Autodesk Fusion 360 part; units mm, degrees
(part 3 of 8)
  spline S62 degree 5 poles (147.1509, -702.208) (147.1492, -702.1152) (147.1456, -701.9297) (147.1398, -701.6516) (147.1309, -701.281) (147.1182, -700.8181) (147.1039, -700.3557) (147.0878, -699.8936) (147.0701, -699.4319) (147.0506, -698.9707) (147.0295, -698.5098) (147.0066, -698.0494) (146.982, -697.5895) (146.9557, -697.13) (146.9276, -696.6709) (146.8978, -696.2123) (146.8662, -695.7542) (146.8328, -695.2965) (146.7976, -694.8394) (146.7606, -694.3827) (146.7218, -693.9266) (146.6811, -693.4709) (146.6386, -693.0158) (146.5943, -692.5612) (146.548, -692.1072) (146.4999, -691.6537) (146.4499, -691.2007) (146.3979, -690.7484) (146.344, -690.2966) (146.2882, -689.8455) (146.2303, -689.3949) (146.1705, -688.945) (146.1087, -688.4957) (146.0448, -688.047) (145.9789, -687.599) (145.911, -687.1517) (145.8409, -686.7051) (145.7687, -686.2591) (145.6944, -685.8139) (145.6179, -685.3695) (145.5392, -684.9257) (145.4583, -684.4828) (145.3751, -684.0406) (145.2897, -683.5993) (145.202, -683.1587) (145.1119, -682.719) (145.0195, -682.2802) (144.9245, -681.8423) (144.8271, -681.4053) (144.7272, -680.9693) (144.6248, -680.5342) (144.5198, -680.1001) (144.4122, -679.667) (144.3019, -679.2349) (144.1889, -678.804) (144.073, -678.3742) (143.9541, -677.9456) (143.8321, -677.5183) (143.7069, -677.0924) (143.5786, -676.6678) (143.447, -676.2445) (143.3123, -675.8226) (143.1743, -675.4021) (143.0469, -675.0245) (142.9454, -674.7318) (142.8716, -674.5233) (142.8267, -674.3982) (142.8115, -674.3563) knots -1 -1 -1 -1 -1 -1 -0.98571429 -0.97142857 -0.95714286 -0.94285714 -0.92857143 -0.91428571 -0.9 -0.88571429 -0.87142857 -0.85714286 -0.84285714 -0.82857143 -0.81428571 -0.8 -0.78571429 -0.77142857 -0.75714286 -0.74285714 -0.72857143 -0.71428571 -0.7 -0.68571429 -0.67142857 -0.65714286 -0.64285714 -0.62857143 -0.61428571 -0.6 -0.58571429 -0.57142857 -0.55714286 -0.54285714 -0.52857143 -0.51428571 -0.5 -0.48571429 -0.47142857 -0.45714286 -0.44285714 -0.42857143 -0.41428571 -0.4 -0.38571429 -0.37142857 -0.35714286 -0.34285714 -0.32857143 -0.31428571 -0.3 -0.28571429 -0.27142857 -0.25714286 -0.24285714 -0.22857143 -0.21428571 -0.2 -0.18571429 -0.17142857 -0.15714286 -0.14285714 -0.12857143 -0.11428571 -0.10707295 -0.10707295 -0.10707295 -0.10707295 -0.10707295 -0.10707295
  spline S63 degree 3 poles (143.5326, -672.4308) (143.352, -672.5314) (143.1927, -672.6663) (142.935, -672.9895) (142.8388, -673.1747) (142.7342, -673.5335) (142.713, -673.7002) (142.7234, -674.0341) (142.7549, -674.1991) (142.8115, -674.3563) knots 0 0 0 0 0.062015 0.062015 0.12403 0.12403 0.174133 0.174133 0.224236 0.224236 0.224236 0.224236
  arc A32 (143.5326, -672.4308) -> (150.7922, -668.2395) centre (11.949, -436.1388) ccw
  spline S64 degree 3 poles (152.8201, -668.5778) (152.6868, -668.4198) (152.5239, -668.2894) (152.1572, -668.0984) (151.957, -668.0397) (151.5848, -668.0058) (151.4171, -668.017) (151.0914, -668.0912) (150.9355, -668.1538) (150.7922, -668.2395) knots 0 0 0 0 0.062015 0.062015 0.12403 0.12403 0.174133 0.174133 0.224236 0.224236 0.224236 0.224236
  spline S65 degree 5 poles (152.8201, -668.5778) (152.8489, -668.6118) (152.9348, -668.7133) (153.0785, -668.8815) (153.2812, -669.1158) (153.5444, -669.4149) (153.8396, -669.7446) (154.1377, -670.0723) (154.4385, -670.3978) (154.742, -670.7213) (155.0483, -671.0427) (155.3573, -671.362) (155.669, -671.6792) (155.9833, -671.9945) (156.3, -672.3078) (156.6191, -672.6194) (156.9403, -672.9291) (157.2638, -673.2371) (157.5893, -673.5433) (157.917, -673.8479) (158.2467, -674.1507) (158.5785, -674.4519) (158.9123, -674.7514) (159.2481, -675.0492) (159.5857, -675.3455) (159.9252, -675.6401) (160.2666, -675.9332) (160.6098, -676.2247) (160.9547, -676.5148) (161.3014, -676.8032) (161.6497, -677.0902) (161.9998, -677.3757) (162.3516, -677.6597) (162.705, -677.9422) (163.06, -678.2233) (163.4167, -678.5029) (163.7748, -678.7811) (164.1346, -679.0579) (164.4959, -679.3332) (164.8587, -679.6072) (165.223, -679.8797) (165.5887, -680.1509) (165.956, -680.4207) (166.3246, -680.6891) (166.6947, -680.9562) (167.0662, -681.2219) (167.4391, -681.4863) (167.8134, -681.7493) (168.189, -682.011) (168.566, -682.2714) (168.9443, -682.5304) (169.324, -682.7882) (169.7049, -683.0446) (170.0871, -683.2998) (170.4707, -683.5536) (170.8555, -683.8062) (171.2415, -684.0574) (171.6288, -684.3074) (172.0173, -684.5562) (172.407, -684.8036) (172.798, -685.0498) (173.1901, -685.2947) (173.5835, -685.5384) (173.978, -685.7809) (174.2945, -685.9738) (174.5324, -686.118) (174.6913, -686.2138) (174.7708, -686.2617) knots 0.10707295 0.10707295 0.10707295 0.10707295 0.10707295 0.10707295 0.11428571 0.12857143 0.14285714 0.15714286 0.17142857 0.18571429 0.2 0.21428571 0.22857143 0.24285714 0.25714286 0.27142857 0.28571429 0.3 0.31428571 0.32857143 0.34285714 0.35714286 0.37142857 0.38571429 0.4 0.41428571 0.42857143 0.44285714 0.45714286 0.47142857 0.48571429 0.5 0.51428571 0.52857143 0.54285714 0.55714286 0.57142857 0.58571429 0.6 0.61428571 0.62857143 0.64285714 0.65714286 0.67142857 0.68571429 0.7 0.71428571 0.72857143 0.74285714 0.75714286 0.77142857 0.78571429 0.8 0.81428571 0.82857143 0.84285714 0.85714286 0.87142857 0.88571429 0.9 0.91428571 0.92857143 0.94285714 0.95714286 0.97142857 0.98571429 1 1 1 1 1 1
  arc A33 (174.7708, -686.2617) -> (182.8648, -680.8022) centre (11.949, -436.1388) ccw
  spline S66 degree 5 poles (182.8648, -680.8022) (182.8502, -680.7106) (182.8208, -680.5274) (182.7763, -680.2527) (182.716, -679.887) (182.639, -679.4304) (182.5604, -678.9744) (182.4802, -678.5191) (182.3984, -678.0644) (182.315, -677.6103) (182.2299, -677.1569) (182.1432, -676.7042) (182.0548, -676.2521) (181.9648, -675.8007) (181.8731, -675.35) (181.7797, -674.9) (181.6847, -674.4508) (181.5879, -674.0022) (181.4894, -673.5544) (181.3892, -673.1073) (181.2873, -672.661) (181.1836, -672.2155) (181.0782, -671.7707) (180.971, -671.3267) (180.862, -670.8835) (180.7513, -670.4411) (180.6387, -669.9996) (180.5243, -669.5589) (180.408, -669.119) (180.2899, -668.68) (180.17, -668.2419) (180.0481, -667.8046) (179.9244, -667.3683) (179.7987, -666.9329) (179.6711, -666.4985) (179.5415, -666.0649) (179.41, -665.6324) (179.2764, -665.2009) (179.1409, -664.7704) (179.0032, -664.3409) (178.8636, -663.9124) (178.7218, -663.485) (178.5779, -663.0587) (178.4319, -662.6335) (178.2837, -662.2095) (178.1333, -661.7866) (177.9807, -661.3649) (177.8258, -660.9445) (177.6685, -660.5253) (177.5089, -660.1074) (177.3469, -659.6908) (177.1825, -659.2756) (177.0157, -658.8617) (176.8463, -658.4492) (176.6744, -658.0381) (176.4998, -657.6287) (176.3225, -657.2208) (176.1422, -656.8147) (175.9589, -656.4103) (175.7727, -656.0077) (175.5836, -655.6068) (175.3914, -655.2078) (175.1963, -654.8105) (175.0176, -654.4544) (174.8763, -654.1787) (174.7741, -653.9824) (174.7123, -653.8648) (174.6915, -653.8254) knots -1 -1 -1 -1 -1 -1 -0.98571429 -0.97142857 -0.95714286 -0.94285714 -0.92857143 -0.91428571 -0.9 -0.88571429 -0.87142857 -0.85714286 -0.84285714 -0.82857143 -0.81428571 -0.8 -0.78571429 -0.77142857 -0.75714286 -0.74285714 -0.72857143 -0.71428571 -0.7 -0.68571429 -0.67142857 -0.65714286 -0.64285714 -0.62857143 -0.61428571 -0.6 -0.58571429 -0.57142857 -0.55714286 -0.54285714 -0.52857143 -0.51428571 -0.5 -0.48571429 -0.47142857 -0.45714286 -0.44285714 -0.42857143 -0.41428571 -0.4 -0.38571429 -0.37142857 -0.35714286 -0.34285714 -0.32857143 -0.31428571 -0.3 -0.28571429 -0.27142857 -0.25714286 -0.24285714 -0.22857143 -0.21428571 -0.2 -0.18571429 -0.17142857 -0.15714286 -0.14285714 -0.12857143 -0.11428571 -0.10707295 -0.10707295 -0.10707295 -0.10707295 -0.10707295 -0.10707295
  spline S67 degree 3 poles (175.1375, -651.8184) (174.9727, -651.9431) (174.8338, -652.0988) (174.6235, -652.4548) (174.5541, -652.6516) (174.5004, -653.0214) (174.5026, -653.1895) (174.5593, -653.5186) (174.6135, -653.6777) (174.6915, -653.8254) knots 0 0 0 0 0.062015 0.062015 0.12403 0.12403 0.174133 0.174133 0.224236 0.224236 0.224236 0.224236
  arc A34 (175.1375, -651.8184) -> (181.7431, -646.6575) centre (11.949, -436.1388) ccw
  spline S68 degree 3 poles (183.7985, -646.7102) (183.6444, -646.5724) (183.4649, -646.4659) (183.0753, -646.3278) (182.8688, -646.2975) (182.4955, -646.3157) (182.331, -646.3501) (182.0189, -646.469) (181.8731, -646.5526) (181.7431, -646.6575) knots 0 0 0 0 0.062015 0.062015 0.12403 0.12403 0.174133 0.174133 0.224236 0.224236 0.224236 0.224236
  spline S69 degree 5 poles (183.7985, -646.7102) (183.8317, -646.74) (183.9308, -646.8284) (184.0965, -646.9751) (184.3299, -647.1788) (184.6322, -647.4384) (184.9704, -647.7239) (185.3112, -648.0068) (185.6543, -648.2873) (185.9999, -648.5654) (186.348, -648.841) (186.6984, -649.1142) (187.0513, -649.385) (187.4063, -649.6535) (187.7636, -649.9197) (188.1229, -650.1838) (188.4841, -650.4458) (188.8473, -650.7058) (189.2123, -650.9637) (189.5792, -651.2197) (189.9478, -651.4737) (190.3183, -651.7257) (190.6905, -651.9759) (191.0645, -652.2241) (191.4401, -652.4705) (191.8173, -652.715) (192.1961, -652.9577) (192.5765, -653.1987) (192.9584, -653.4378) (193.3419, -653.6753) (193.7268, -653.911) (194.1132, -654.145) (194.5011, -654.3772) (194.8904, -654.6078) (195.2811, -654.8367) (195.6731, -655.064) (196.0666, -655.2897) (196.4613, -655.5137) (196.8574, -655.7361) (197.2548, -655.9568) (197.6535, -656.1761) (198.0534, -656.3937) (198.4546, -656.6097) (198.8571, -656.8242) (199.2607, -657.0372) (199.6656, -657.2486) (200.0717, -657.4585) (200.4789, -657.6669) (200.8873, -657.8738) (201.2969, -658.0792) (201.7076, -658.283) (202.1194, -658.4854) (202.5323, -658.6864) (202.9463, -658.8858) (203.3614, -659.0838) (203.7776, -659.2804) (204.1949, -659.4755) (204.6132, -659.6691) (205.0326, -659.8614) (205.4529, -660.0522) (205.8743, -660.2416) (206.2968, -660.4295) (206.7202, -660.6161) (207.1446, -660.8013) (207.4849, -660.9483) (207.7406, -661.0579) (207.9112, -661.1307) (207.9966, -661.1671) knots 0.10707295 0.10707295 0.10707295 0.10707295 0.10707295 0.10707295 0.11428571 0.12857143 0.14285714 0.15714286 0.17142857 0.18571429 0.2 0.21428571 0.22857143 0.24285714 0.25714286 0.27142857 0.28571429 0.3 0.31428571 0.32857143 0.34285714 0.35714286 0.37142857 0.38571429 0.4 0.41428571 0.42857143 0.44285714 0.45714286 0.47142857 0.48571429 0.5 0.51428571 0.52857143 0.54285714 0.55714286 0.57142857 0.58571429 0.6 0.61428571 0.62857143 0.64285714 0.65714286 0.67142857 0.68571429 0.7 0.71428571 0.72857143 0.74285714 0.75714286 0.77142857 0.78571429 0.8 0.81428571 0.82857143 0.84285714 0.85714286 0.87142857 0.88571429 0.9 0.91428571 0.92857143 0.94285714 0.95714286 0.97142857 0.98571429 1 1 1 1 1 1
  arc A35 (207.9966, -661.1671) -> (215.252, -654.6343) centre (11.949, -436.1388) ccw
  spline S70 degree 5 poles (215.252, -654.6343) (215.2248, -654.5455) (215.1703, -654.3682) (215.0879, -654.1025) (214.9773, -653.7486) (214.8375, -653.3072) (214.6962, -652.8666) (214.5534, -652.4269) (214.4091, -651.988) (214.2633, -651.55) (214.116, -651.1128) (213.9671, -650.6765) (213.8167, -650.2412) (213.6647, -649.8067) (213.5112, -649.3732) (213.3561, -648.9406) (213.1994, -648.5089) (213.0412, -648.0782) (212.8814, -647.6484) (212.7199, -647.2197) (212.5569, -646.7919) (212.3922, -646.3651) (212.2259, -645.9393) (212.0579, -645.5146) (211.8883, -645.0909) (211.7171, -644.6682) (211.5441, -644.2466) (211.3695, -643.8261) (211.1932, -643.4067) (211.0151, -642.9884) (210.8354, -642.5712) (210.6538, -642.1552) (210.4706, -641.7404) (210.2855, -641.3267) (210.0987, -640.9142) (209.9101, -640.503) (209.7196, -640.0929) (209.5273, -639.6842) (209.3331, -639.2767) (209.1371, -638.8706) (208.9391, -638.4657) (208.7393, -638.0622) (208.5375, -637.6601) (208.3337, -637.2594) (208.1279, -636.8601) (207.9202, -636.4622) (207.7103, -636.0659) (207.4984, -635.6711) (207.2843, -635.2779) (207.0681, -634.8863) (206.8497, -634.4963) (206.6291, -634.108) (206.4063, -633.7213) (206.1812, -633.3364) (205.9538, -632.9533) (205.7239, -632.5721) (205.4915, -632.1929) (205.2564, -631.8158) (205.0187, -631.4408) (204.7783, -631.0681) (204.5351, -630.6975) (204.2894, -630.329) (204.0408, -629.9628) (203.8142, -629.635) (203.636, -629.3816) (203.5075, -629.2015) (203.4299, -629.0937) (203.4038, -629.0575) knots -1 -1 -1 -1 -1 -1 -0.98571429 -0.97142857 -0.95714286 -0.94285714 -0.92857143 -0.91428571 -0.9 -0.88571429 -0.87142857 -0.85714286 -0.84285714 -0.82857143 -0.81428571 -0.8 -0.78571429 -0.77142857 -0.75714286 -0.74285714 -0.72857143 -0.71428571 -0.7 -0.68571429 -0.67142857 -0.65714286 -0.64285714 -0.62857143 -0.61428571 -0.6 -0.58571429 -0.57142857 -0.55714286 -0.54285714 -0.52857143 -0.51428571 -0.5 -0.48571429 -0.47142857 -0.45714286 -0.44285714 -0.42857143 -0.41428571 -0.4 -0.38571429 -0.37142857 -0.35714286 -0.34285714 -0.32857143 -0.31428571 -0.3 -0.28571429 -0.27142857 -0.25714286 -0.24285714 -0.22857143 -0.21428571 -0.2 -0.18571429 -0.17142857 -0.15714286 -0.14285714 -0.12857143 -0.11428571 -0.10707295 -0.10707295 -0.10707295 -0.10707295 -0.10707295 -0.10707295
  spline S71 degree 3 poles (203.5662, -627.0079) (203.4203, -627.1544) (203.3044, -627.3279) (203.1457, -627.7097) (203.1044, -627.9142) (203.1026, -628.288) (203.1282, -628.454) (203.2302, -628.7721) (203.306, -628.9221) (203.4038, -629.0575) knots 0 0 0 0 0.062015 0.062015 0.12403 0.12403 0.174133 0.174133 0.224236 0.224236 0.224236 0.224236
  arc A36 (203.5662, -627.0079) -> (209.3892, -620.978) centre (11.949, -436.1388) ccw
  spline S72 degree 3 poles (211.4319, -620.7441) (211.2602, -620.6291) (211.0676, -620.5486) (210.6625, -620.4661) (210.4538, -620.4648) (210.0867, -620.5348) (209.9286, -620.5918) (209.6361, -620.7529) (209.5034, -620.856) (209.3892, -620.978) knots 0 0 0 0 0.062015 0.062015 0.12403 0.12403 0.174133 0.174133 0.224236 0.224236 0.224236 0.224236
  spline S73 degree 5 poles (211.4319, -620.7441) (211.4689, -620.769) (211.5794, -620.8428) (211.7639, -620.9649) (212.0234, -621.1342) (212.3589, -621.3492) (212.7335, -621.5848) (213.1103, -621.8176) (213.4892, -622.0476) (213.8702, -622.2749) (214.2532, -622.4994) (214.6382, -622.7211) (215.0253, -622.9402) (215.4143, -623.1566) (215.8051, -623.3705) (216.1977, -623.582) (216.5919, -623.7912) (216.9877, -623.9981) (217.385, -624.2028) (217.784, -624.4052) (218.1844, -624.6054) (218.5863, -624.8035) (218.9897, -624.9993) (219.3946, -625.1931) (219.8008, -625.3848) (220.2084, -625.5745) (220.6173, -625.7621) (221.0276, -625.9478) (221.4391, -626.1315) (221.8518, -626.3132) (222.2658, -626.493) (222.681, -626.671) (223.0974, -626.847) (223.515, -627.0212) (223.9338, -627.1935) (224.3537, -627.364) (224.7747, -627.5327) (225.1968, -627.6996) (225.6199, -627.8647) (226.0442, -628.028) (226.4695, -628.1896) (226.8958, -628.3494) (227.3232, -628.5076) (227.7516, -628.664) (228.181, -628.8187) (228.6113, -628.9717) (229.0426, -629.123) (229.4749, -629.2727) (229.9081, -629.4207) (230.3423, -629.5671) (230.7773, -629.7119) (231.2133, -629.855) (231.6502, -629.9965) (232.0879, -630.1364) (232.5266, -630.2747) (232.9661, -630.4114) (233.4064, -630.5465) (233.8476, -630.6801) (234.2897, -630.8121) (234.7325, -630.9425) (235.1762, -631.0714) (235.6206, -631.1988) (236.0659, -631.3246) (236.5119, -631.4489) (236.8694, -631.5471) (237.1378, -631.6201) (237.317, -631.6685) (237.4066, -631.6926) knots 0.10707295 0.10707295 0.10707295 0.10707295 0.10707295 0.10707295 0.11428571 0.12857143 0.14285714 0.15714286 0.17142857 0.18571429 0.2 0.21428571 0.22857143 0.24285714 0.25714286 0.27142857 0.28571429 0.3 0.31428571 0.32857143 0.34285714 0.35714286 0.37142857 0.38571429 0.4 0.41428571 0.42857143 0.44285714 0.45714286 0.47142857 0.48571429 0.5 0.51428571 0.52857143 0.54285714 0.55714286 0.57142857 0.58571429 0.6 0.61428571 0.62857143 0.64285714 0.65714286 0.67142857 0.68571429 0.7 0.71428571 0.72857143 0.74285714 0.75714286 0.77142857 0.78571429 0.8 0.81428571 0.82857143 0.84285714 0.85714286 0.87142857 0.88571429 0.9 0.91428571 0.92857143 0.94285714 0.95714286 0.97142857 0.98571429 1 1 1 1 1 1
  arc A37 (237.4066, -631.6926) -> (243.6822, -624.2136) centre (11.949, -436.1388) ccw
  spline S74 degree 5 poles (243.6822, -624.2136) (243.6429, -624.1295) (243.5642, -623.9615) (243.4457, -623.7098) (243.2869, -623.3748) (243.087, -622.9571) (242.8858, -622.5405) (242.6832, -622.1249) (242.4792, -621.7104) (242.2739, -621.2969) (242.0671, -620.8845) (241.859, -620.4732) (241.6494, -620.063) (241.4385, -619.6539) (241.2261, -619.246) (241.0123, -618.8391) (240.7971, -618.4335) (240.5804, -618.029) (240.3624, -617.6257) (240.1428, -617.2235) (239.9218, -616.8226) (239.6993, -616.4229) (239.4754, -616.0244) (239.25, -615.6271) (239.0231, -615.2312) (238.7946, -614.8365) (238.5647, -614.443) (238.3333, -614.0509) (238.1003, -613.6601) (237.8657, -613.2707) (237.6297, -612.8826) (237.392, -612.4959) (237.1528, -612.1106) (236.912, -611.7267) (236.6695, -611.3442) (236.4255, -610.9632) (236.1798, -610.5837) (235.9325, -610.2057) (235.6835, -609.8292) (235.4329, -609.4543) (235.1805, -609.081) (234.9264, -608.7092) (234.6706, -608.3391) (234.4131, -607.9706) (234.1537, -607.6038) (233.8926, -607.2388) (233.6297, -606.8755) (233.3648, -606.5141) (233.0981, -606.1545) (232.8295, -605.7968) (232.5589, -605.441) (232.2865, -605.0871) (232.012, -604.7352) (231.7355, -604.3854) (231.457, -604.0377) (231.1763, -603.6922) (230.8934, -603.349) (230.6081, -603.0083) (230.3205, -602.6701) (230.0306, -602.3344) (229.7382, -602.0012) (229.4436, -601.6706) (229.1465, -601.3425) (228.8765, -601.0494) (228.6647, -600.8233) (228.5124, -600.6628) (228.4205, -600.5668) (228.3897, -600.5347) knots -1 -1 -1 -1 -1 -1 -0.98571429 -0.97142857 -0.95714286 -0.94285714 -0.92857143 -0.91428571 -0.9 -0.88571429 -0.87142857 -0.85714286 -0.84285714 -0.82857143 -0.81428571 -0.8 -0.78571429 -0.77142857 -0.75714286 -0.74285714 -0.72857143 -0.71428571 -0.7 -0.68571429 -0.67142857 -0.65714286 -0.64285714 -0.62857143 -0.61428571 -0.6 -0.58571429 -0.57142857 -0.55714286 -0.54285714 -0.52857143 -0.51428571 -0.5 -0.48571429 -0.47142857 -0.45714286 -0.44285714 -0.42857143 -0.41428571 -0.4 -0.38571429 -0.37142857 -0.35714286 -0.34285714 -0.32857143 -0.31428571 -0.3 -0.28571429 -0.27142857 -0.25714286 -0.24285714 -0.22857143 -0.21428571 -0.2 -0.18571429 -0.17142857 -0.15714286 -0.14285714 -0.12857143 -0.11428571 -0.10707295 -0.10707295 -0.10707295 -0.10707295 -0.10707295 -0.10707295
  spline S75 degree 3 poles (228.2652, -598.4824) (228.1411, -598.6478) (228.0505, -598.8358) (227.9465, -599.2359) (227.934, -599.4442) (227.9844, -599.8145) (228.0328, -599.9754) (228.1781, -600.2762) (228.274, -600.4142) (228.3897, -600.5347) knots 0 0 0 0 0.062015 0.062015 0.12403 0.12403 0.174133 0.174133 0.224236 0.224236 0.224236 0.224236
  arc A38 (228.2652, -598.4824) -> (233.1924, -591.7008) centre (11.949, -436.1388) ccw
  spline S76 degree 3 poles (235.1827, -591.1849) (234.9966, -591.0949) (234.7947, -591.042) (234.3821, -591.0167) (234.1752, -591.0444) (233.8214, -591.1648) (233.6728, -591.2432) (233.4055, -591.4435) (233.2885, -591.5641) (233.1924, -591.7008) knots 0 0 0 0 0.062015 0.062015 0.12403 0.12403 0.174133 0.174133 0.224236 0.224236 0.224236 0.224236
  spline S77 degree 5 poles (235.1827, -591.1849) (235.2228, -591.2043) (235.3425, -591.2621) (235.5422, -591.3573) (235.8227, -591.4889) (236.1848, -591.6551) (236.5886, -591.8362) (236.9941, -592.0143) (237.4014, -592.1894) (237.8102, -592.3614) (238.2207, -592.5304) (238.6329, -592.6964) (239.0467, -592.8595) (239.4621, -593.0197) (239.8788, -593.1771) (240.297, -593.3319) (240.7165, -593.4842) (241.1372, -593.634) (241.5592, -593.7814) (241.9824, -593.9263) (242.4068, -594.0689) (242.8324, -594.209) (243.2592, -594.3469) (243.687, -594.4824) (244.116, -594.6157) (244.546, -594.7468) (244.9771, -594.8757) (245.4091, -595.0024) (245.8422, -595.1271) (246.2762, -595.2496) (246.7112, -595.3701) (247.1472, -595.4885) (247.584, -595.6049) (248.0218, -595.7192) (248.4604, -595.8316) (248.9, -595.942) (249.3403, -596.0504) (249.7816, -596.157) (250.2236, -596.2616) (250.6665, -596.3643) (251.1101, -596.4651) (251.5546, -596.564) (251.9998, -596.6612) (252.4457, -596.7564) (252.8925, -596.8499) (253.3399, -596.9415) (253.7881, -597.0313) (254.237, -597.1194) (254.6866, -597.2057) (255.1369, -597.2902) (255.5879, -597.373) (256.0395, -597.4541) (256.4919, -597.5334) (256.9448, -597.611) (257.3984, -597.6869) (257.8527, -597.7611) (258.3076, -597.8336) (258.763, -597.9045) (259.2191, -597.9737) (259.6758, -598.0412) (260.1331, -598.1071) (260.591, -598.1714) (261.0494, -598.234) (261.5084, -598.2951) (261.8761, -598.3426) (262.1521, -598.3775) (262.3362, -598.4004) (262.4283, -598.4118) knots 0.10707295 0.10707295 0.10707295 0.10707295 0.10707295 0.10707295 0.11428571 0.12857143 0.14285714 0.15714286 0.17142857 0.18571429 0.2 0.21428571 0.22857143 0.24285714 0.25714286 0.27142857 0.28571429 0.3 0.31428571 0.32857143 0.34285714 0.35714286 0.37142857 0.38571429 0.4 0.41428571 0.42857143 0.44285714 0.45714286 0.47142857 0.48571429 0.5 0.51428571 0.52857143 0.54285714 0.55714286 0.57142857 0.58571429 0.6 0.61428571 0.62857143 0.64285714 0.65714286 0.67142857 0.68571429 0.7 0.71428571 0.72857143 0.74285714 0.75714286 0.77142857 0.78571429 0.8 0.81428571 0.82857143 0.84285714 0.85714286 0.87142857 0.88571429 0.9 0.91428571 0.92857143 0.94285714 0.95714286 0.97142857 0.98571429 1 1 1 1 1 1
  arc A39 (262.4283, -598.4118) -> (267.6019, -590.1322) centre (11.949, -436.1388) ccw
  spline S78 degree 5 poles (267.6019, -590.1322) (267.5513, -590.0544) (267.45, -589.899) (267.2976, -589.6662) (267.0938, -589.3566) (266.8377, -588.9708) (266.5804, -588.5862) (266.322, -588.2029) (266.0623, -587.8208) (265.8014, -587.4399) (265.5392, -587.0603) (265.2759, -586.682) (265.0113, -586.3049) (264.7455, -585.9292) (264.4784, -585.5548) (264.2101, -585.1817) (263.9405, -584.8099) (263.6696, -584.4395) (263.3975, -584.0705) (263.1242, -583.7028) (262.8495, -583.3365) (262.5736, -582.9716) (262.2964, -582.6082) (262.0179, -582.2462) (261.738, -581.8857) (261.4569, -581.5266) (261.1745, -581.169) (260.8907, -580.8129) (260.6056, -580.4584) (260.3191, -580.1053) (260.0313, -579.7539) (259.7422, -579.404) (259.4517, -579.0557) (259.1598, -578.7091) (258.8665, -578.3641) (258.5718, -578.0208) (258.2757, -577.6791) (257.9782, -577.3392) (257.6792, -577.0011) (257.3788, -576.6647) (257.0769, -576.3301) (256.7736, -575.9973) (256.4688, -575.6664) (256.1624, -575.3373) (255.8546, -575.0102) (255.5452, -574.6851) (255.2342, -574.3619) (254.9217, -574.0409) (254.6075, -573.7219) (254.2917, -573.4051) (253.9743, -573.0904) (253.6552, -572.7779) (253.3345, -572.4676) (253.012, -572.1597) (252.6878, -571.8541) (252.3617, -571.551) (252.0338, -571.2506) (251.7039, -570.9529) (251.372, -570.658) (251.0382, -570.3659) (250.7023, -570.0766) (250.3645, -569.7902) (250.0246, -569.5067) (249.7165, -569.2541) (249.4753, -569.0596) (249.3022, -568.9219) (249.1978, -568.8396) (249.1628, -568.8121) knots -1 -1 -1 -1 -1 -1 -0.98571429 -0.97142857 -0.95714286 -0.94285714 -0.92857143 -0.91428571 -0.9 -0.88571429 -0.87142857 -0.85714286 -0.84285714 -0.82857143 -0.81428571 -0.8 -0.78571429 -0.77142857 -0.75714286 -0.74285714 -0.72857143 -0.71428571 -0.7 -0.68571429 -0.67142857 -0.65714286 -0.64285714 -0.62857143 -0.61428571 -0.6 -0.58571429 -0.57142857 -0.55714286 -0.54285714 -0.52857143 -0.51428571 -0.5 -0.48571429 -0.47142857 -0.45714286 -0.44285714 -0.42857143 -0.41428571 -0.4 -0.38571429 -0.37142857 -0.35714286 -0.34285714 -0.32857143 -0.31428571 -0.3 -0.28571429 -0.27142857 -0.25714286 -0.24285714 -0.22857143 -0.21428571 -0.2 -0.18571429 -0.17142857 -0.15714286 -0.14285714 -0.12857143 -0.11428571 -0.10707295 -0.10707295 -0.10707295 -0.10707295 -0.10707295 -0.10707295
  spline S79 degree 3 poles (248.7539, -566.7971) (248.6541, -566.9781) (248.5905, -567.1769) (248.5432, -567.5876) (248.5598, -567.7956) (248.6612, -568.1553) (248.7316, -568.3079) (248.9173, -568.5856) (249.0315, -568.7089) (249.1628, -568.8121) knots 0 0 0 0 0.062015 0.062015 0.12403 0.12403 0.174133 0.174133 0.224236 0.224236 0.224236 0.224236
  arc A40 (248.7539, -566.7971) -> (252.6893, -559.3957) centre (11.949, -436.1388) ccw
  spline S80 degree 3 poles (254.5884, -558.6079) (254.3916, -558.5446) (254.1844, -558.5204) (253.7722, -558.5527) (253.5712, -558.609) (253.2376, -558.7774) (253.1014, -558.8758) (252.8645, -559.1113) (252.7654, -559.247) (252.6893, -559.3957) knots 0 0 0 0 0.062015 0.062015 0.12403 0.12403 0.174133 0.174133 0.224236 0.224236 0.224236 0.224236
  spline S81 degree 5 poles (254.5884, -558.6079) (254.6309, -558.6216) (254.7574, -558.6621) (254.9684, -558.7286) (255.2645, -558.8198) (255.6462, -558.934) (256.0713, -559.0572) (256.4977, -559.1771) (256.9253, -559.2938) (257.3541, -559.4073) (257.7842, -559.5175) (258.2155, -559.6245) (258.6479, -559.7284) (259.0815, -559.8292) (259.5162, -559.9271) (259.9518, -560.0222) (260.3884, -560.1147) (260.8259, -560.2045) (261.2643, -560.2916) (261.7035, -560.3763) (262.1436, -560.4584) (262.5846, -560.5379) (263.0264, -560.615) (263.4689, -560.6897) (263.9123, -560.762) (264.3564, -560.832) (264.8012, -560.8996) (265.2467, -560.965) (265.6929, -561.0282) (266.1397, -561.0891) (266.5873, -561.1479) (267.0354, -561.2045) (267.4842, -561.2589) (267.9337, -561.3112) (268.3837, -561.3614) (268.8343, -561.4096) (269.2855, -561.4557) (269.7372, -561.4998) (270.1895, -561.5418) (270.6424, -561.5819) (271.0957, -561.62) (271.5496, -561.6562) (272.004, -561.6903) (272.4589, -561.7226) (272.9143, -561.753) (273.3701, -561.7815) (273.8265, -561.808) (274.2833, -561.8328) (274.7405, -561.8557) (275.1982, -561.8767) (275.6563, -561.8959) (276.1148, -561.9133) (276.5738, -561.9289) (277.0331, -561.9427) (277.4929, -561.9548) (277.953, -561.965) (278.4136, -561.9736) (278.8745, -561.9803) (279.3358, -561.9854) (279.7974, -561.9887) (280.2594, -561.9903) (280.7218, -561.9902) (281.1845, -561.9885) (281.6475, -561.985) (282.0182, -561.9809) (282.2964, -561.977) (282.4819, -561.9741) (282.5747, -561.9726) knots 0.10707295 0.10707295 0.10707295 0.10707295 0.10707295 0.10707295 0.11428571 0.12857143 0.14285714 0.15714286 0.17142857 0.18571429 0.2 0.21428571 0.22857143 0.24285714 0.25714286 0.27142857 0.28571429 0.3 0.31428571 0.32857143 0.34285714 0.35714286 0.37142857 0.38571429 0.4 0.41428571 0.42857143 0.44285714 0.45714286 0.47142857 0.48571429 0.5 0.51428571 0.52857143 0.54285714 0.55714286 0.57142857 0.58571429 0.6 0.61428571 0.62857143 0.64285714 0.65714286 0.67142857 0.68571429 0.7 0.71428571 0.72857143 0.74285714 0.75714286 0.77142857 0.78571429 0.8 0.81428571 0.82857143 0.84285714 0.85714286 0.87142857 0.88571429 0.9 0.91428571 0.92857143 0.94285714 0.95714286 0.97142857 0.98571429 1 1 1 1 1 1
  arc A41 (282.5747, -561.9726) -> (286.5457, -553.0535) centre (11.949, -436.1388) ccw
  spline S82 degree 5 poles (286.5457, -553.0535) (286.4848, -552.9836) (286.3628, -552.8438) (286.1795, -552.6345) (285.9345, -552.3562) (285.6273, -552.0098) (285.319, -551.6648) (285.0097, -551.3211) (284.6993, -550.9789) (284.388, -550.638) (284.0755, -550.2986) (283.7621, -549.9606) (283.4476, -549.6241) (283.1321, -549.289) (282.8155, -548.9554) (282.4978, -548.6232) (282.1791, -548.2926) (281.8594, -547.9635) (281.5386, -547.6359) (281.2167, -547.3099) (280.8937, -546.9854) (280.5697, -546.6625) (280.2446, -546.3412) (279.9184, -546.0214) (279.5912, -545.7033) (279.2628, -545.3869) (278.9333, -545.0721) (278.6028, -544.759) (278.2711, -544.4475) (277.9383, -544.1378) (277.6044, -543.8298) (277.2693, -543.5236) (276.9332, -543.2192) (276.5959, -542.9165) (276.2574, -542.6157) (275.9178, -542.3167) (275.5771, -542.0196) (275.2351, -541.7244) (274.892, -541.4312) (274.5477, -541.1399) (274.2022, -540.8505) (273.8555, -540.5632) (273.5076, -540.2779) (273.1585, -539.9947) (272.8081, -539.7136) (272.4565, -539.4347) (272.1036, -539.158) (271.7494, -538.8836) (271.3939, -538.6114) (271.037, -538.3416) (270.6789, -538.0742) (270.3194, -537.8091) (269.9586, -537.5465) (269.5964, -537.2864) (269.2328, -537.0289) (268.8678, -536.7742) (268.5012, -536.5223) (268.1331, -536.2734) (267.7634, -536.0276) (267.3922, -535.7848) (267.0193, -535.5451) (266.6449, -535.3085) (266.2689, -535.0751) (265.9286, -534.8678) (265.6628, -534.7088) (265.4721, -534.5965) (265.3573, -534.5295) (265.3188, -534.5071) knots -1 -1 -1 -1 -1 -1 -0.98571429 -0.97142857 -0.95714286 -0.94285714 -0.92857143 -0.91428571 -0.9 -0.88571429 -0.87142857 -0.85714286 -0.84285714 -0.82857143 -0.81428571 -0.8 -0.78571429 -0.77142857 -0.75714286 -0.74285714 -0.72857143 -0.71428571 -0.7 -0.68571429 -0.67142857 -0.65714286 -0.64285714 -0.62857143 -0.61428571 -0.6 -0.58571429 -0.57142857 -0.55714286 -0.54285714 -0.52857143 -0.51428571 -0.5 -0.48571429 -0.47142857 -0.45714286 -0.44285714 -0.42857143 -0.41428571 -0.4 -0.38571429 -0.37142857 -0.35714286 -0.34285714 -0.32857143 -0.31428571 -0.3 -0.28571429 -0.27142857 -0.25714286 -0.24285714 -0.22857143 -0.21428571 -0.2 -0.18571429 -0.17142857 -0.15714286 -0.14285714 -0.12857143 -0.11428571 -0.10707295 -0.10707295 -0.10707295 -0.10707295 -0.10707295 -0.10707295
  spline S83 degree 3 poles (264.6335, -532.5687) (264.5598, -532.7618) (264.5245, -532.9675) (264.5348, -533.3808) (264.5802, -533.5845) (264.7307, -533.9266) (264.8216, -534.0679) (265.0442, -534.317) (265.1744, -534.4232) (265.3188, -534.5071) knots 0 0 0 0 0.062015 0.062015 0.12403 0.12403 0.174133 0.174133 0.224236 0.224236 0.224236 0.224236
  arc A42 (264.6335, -532.5687) -> (267.5005, -524.6916) centre (11.949, -436.1388) ccw
  spline S84 degree 3 poles (269.2715, -523.6472) (269.0678, -523.6119) (268.8592, -523.6167) (268.4555, -523.7061) (268.2643, -523.7898) (267.9574, -524.003) (267.8362, -524.1194) (267.6344, -524.3856) (267.5552, -524.5338) (267.5005, -524.6916) knots 0 0 0 0 0.062015 0.062015 0.12403 0.12403 0.174133 0.174133 0.224236 0.224236 0.224236 0.224236
  spline S85 degree 5 poles (269.2715, -523.6472) (269.3154, -523.6548) (269.4464, -523.6773) (269.6646, -523.7138) (269.9705, -523.7629) (270.3644, -523.8229) (270.8025, -523.8857) (271.2414, -523.9451) (271.6811, -524.0012) (272.1215, -524.0538) (272.5627, -524.1031) (273.0047, -524.1491) (273.4474, -524.1918) (273.8908, -524.2313) (274.3349, -524.2677) (274.7795, -524.3013) (275.2247, -524.3321) (275.6704, -524.3601) (276.1167, -524.3854) (276.5634, -524.4081) (277.0107, -524.4281) (277.4584, -524.4456) (277.9067, -524.4604) (278.3553, -524.4728) (278.8044, -524.4827) (279.2539, -524.4902) (279.7038, -524.4953) (280.154, -524.498) (280.6047, -524.4984) (281.0557, -524.4966) (281.507, -524.4925) (281.9587, -524.4862) (282.4107, -524.4776) (282.8631, -524.4669) (283.3157, -524.454) (283.7686, -524.4389) (284.2218, -524.4218) (284.6753, -524.4026) (285.1291, -524.3813) (285.5831, -524.358) (286.0373, -524.3326) (286.4918, -524.3052) (286.9466, -524.2758) (287.4015, -524.2445) (287.8567, -524.2112) (288.3121, -524.1759) (288.7677, -524.1387) (289.2235, -524.0997) (289.6794, -524.0587) (290.1356, -524.0158) (290.5919, -523.9711) (291.0484, -523.9245) (291.5051, -523.8761) (291.9619, -523.8258) (292.4188, -523.7738) (292.8759, -523.7199) (293.3332, -523.6642) (293.7906, -523.6068) (294.2481, -523.5476) (294.7057, -523.4866) (295.1634, -523.424) (295.6212, -523.3595) (296.0792, -523.2934) (296.5372, -523.2255) (296.9037, -523.1698) (297.1787, -523.1273) (297.362, -523.0986) (297.4536, -523.0842) knots 0.10707295 0.10707295 0.10707295 0.10707295 0.10707295 0.10707295 0.11428571 0.12857143 0.14285714 0.15714286 0.17142857 0.18571429 0.2 0.21428571 0.22857143 0.24285714 0.25714286 0.27142857 0.28571429 0.3 0.31428571 0.32857143 0.34285714 0.35714286 0.37142857 0.38571429 0.4 0.41428571 0.42857143 0.44285714 0.45714286 0.47142857 0.48571429 0.5 0.51428571 0.52857143 0.54285714 0.55714286 0.57142857 0.58571429 0.6 0.61428571 0.62857143 0.64285714 0.65714286 0.67142857 0.68571429 0.7 0.71428571 0.72857143 0.74285714 0.75714286 0.77142857 0.78571429 0.8 0.81428571 0.82857143 0.84285714 0.85714286 0.87142857 0.88571429 0.9 0.91428571 0.92857143 0.94285714 0.95714286 0.97142857 0.98571429 1 1 1 1 1 1
  arc A43 (297.4536, -523.0842) -> (300.1447, -513.6993) centre (11.949, -436.1388) ccw
  spline S86 degree 5 poles (300.1447, -513.6993) (300.0746, -513.6384) (299.9344, -513.517) (299.7238, -513.3352) (299.4424, -513.0938) (299.09, -512.7935) (298.7367, -512.4947) (298.3825, -512.1975) (298.0276, -511.9018) (297.6718, -511.6076) (297.3152, -511.3149) (296.9578, -511.0238) (296.5995, -510.7343) (296.2404, -510.4464) (295.8805, -510.1601) (295.5197, -509.8754) (295.1581, -509.5924) (294.7956, -509.311) (294.4324, -509.0312) (294.0682, -508.7531) (293.7033, -508.4768) (293.3374, -508.2021) (292.9708, -507.9291) (292.6033, -507.6579) (292.2349, -507.3885) (291.8657, -507.1208) (291.4956, -506.8549) (291.1247, -506.5909) (290.7529, -506.3286) (290.3803, -506.0682) (290.0067, -505.8097) (289.6324, -505.5531) (289.2571, -505.2984) (288.8809, -505.0457) (288.5039, -504.7949) (288.126, -504.5461) (287.7472, -504.2993) (287.3675, -504.0545) (286.9869, -503.8119) (286.6054, -503.5713) (286.223, -503.3329) (285.8397, -503.0966) (285.4555, -502.8625) (285.0703, -502.6307) (284.6843, -502.4011) (284.2972, -502.1738) (283.9093, -501.9489) (283.5203, -501.7264) (283.1304, -501.5064) (282.7395, -501.2889) (282.3476, -501.0739) (281.9548, -500.8615) (281.5609, -500.6516) (281.1661, -500.4445) (280.7702, -500.2401) (280.3732, -500.0386) (279.9752, -499.8402) (279.576, -499.645) (279.1757, -499.453) (278.7743, -499.2643) (278.3717, -499.0788) (277.968, -498.8966) (277.5632, -498.7177) (277.1973, -498.5598) (276.9119, -498.4394) (276.7075, -498.3547) (276.5845, -498.3044) (276.5432, -498.2876) knots -1 -1 -1 -1 -1 -1 -0.98571429 -0.97142857 -0.95714286 -0.94285714 -0.92857143 -0.91428571 -0.9 -0.88571429 -0.87142857 -0.85714286 -0.84285714 -0.82857143 -0.81428571 -0.8 -0.78571429 -0.77142857 -0.75714286 -0.74285714 -0.72857143 -0.71428571 -0.7 -0.68571429 -0.67142857 -0.65714286 -0.64285714 -0.62857143 -0.61428571 -0.6 -0.58571429 -0.57142857 -0.55714286 -0.54285714 -0.52857143 -0.51428571 -0.5 -0.48571429 -0.47142857 -0.45714286 -0.44285714 -0.42857143 -0.41428571 -0.4 -0.38571429 -0.37142857 -0.35714286 -0.34285714 -0.32857143 -0.31428571 -0.3 -0.28571429 -0.27142857 -0.25714286 -0.24285714 -0.22857143 -0.21428571 -0.2 -0.18571429 -0.17142857 -0.15714286 -0.14285714 -0.12857143 -0.11428571 -0.10707295 -0.10707295 -0.10707295 -0.10707295 -0.10707295 -0.10707295
  spline S87 degree 3 poles (275.5948, -496.4634) (275.5487, -496.6649) (275.5424, -496.8735) (275.6101, -497.2813) (275.6835, -497.4767) (275.8801, -497.7945) (275.9898, -497.9218) (276.2448, -498.1375) (276.3886, -498.2245) (276.5432, -498.2876) knots 0 0 0 0 0.062015 0.062015 0.12403 0.12403 0.174133 0.174133 0.224236 0.224236 0.224236 0.224236
  arc A44 (275.5948, -496.4634) -> (277.3377, -488.2639) centre (11.949, -436.1388) ccw
  spline S88 degree 3 poles (278.9461, -486.9832) (278.7394, -486.9766) (278.5335, -487.0104) (278.1462, -487.1551) (277.9686, -487.2646) (277.6943, -487.5185) (277.5905, -487.6506) (277.4277, -487.9423) (277.3699, -488.1) (277.3377, -488.2639) knots 0 0 0 0 0.062015 0.062015 0.12403 0.12403 0.174133 0.174133 0.224236 0.224236 0.224236 0.224236
  spline S89 degree 5 poles (278.9461, -486.9832) (278.9906, -486.9846) (279.1234, -486.9886) (279.3446, -486.9944) (279.6543, -487.0005) (280.0528, -487.0051) (280.4954, -487.0063) (280.9383, -487.0041) (281.3815, -486.9984) (281.825, -486.9892) (282.2687, -486.9767) (282.7128, -486.9607) (283.1571, -486.9413) (283.6017, -486.9187) (284.0465, -486.893) (284.4915, -486.8644) (284.9366, -486.8329) (285.3819, -486.7986) (285.8274, -486.7616) (286.273, -486.7218) (286.7186, -486.6794) (287.1645, -486.6344) (287.6104, -486.5867) (288.0564, -486.5365) (288.5025, -486.4838) (288.9486, -486.4287) (289.3949, -486.3711) (289.8411, -486.3112) (290.2874, -486.2489) (290.7338, -486.1843) (291.1802, -486.1174) (291.6266, -486.0483) (292.073, -485.9769) (292.5194, -485.9033) (292.9659, -485.8276) (293.4123, -485.7496) (293.8587, -485.6696) (294.3051, -485.5874) (294.7515, -485.5032) (295.1978, -485.4169) (295.6441, -485.3286) (296.0904, -485.2382) (296.5366, -485.1458) (296.9828, -485.0515) (297.4289, -484.9551) (297.875, -484.8568) (298.3209, -484.7566) (298.7668, -484.6545) (299.2127, -484.5504) (299.6584, -484.4445) (300.1041, -484.3367) (300.5496, -484.2271) (300.9951, -484.1156) (301.4405, -484.0022) (301.8858, -483.8871) (302.3309, -483.7701) (302.776, -483.6513) (303.2209, -483.5308) (303.6657, -483.4085) (304.1104, -483.2845) (304.5549, -483.1587) (304.9994, -483.0312) (305.4436, -482.9019) (305.8878, -482.771) (306.243, -482.6648) (306.5093, -482.5844) (306.6868, -482.5305) (306.7756, -482.5035) knots 0.10707295 0.10707295 0.10707295 0.10707295 0.10707295 0.10707295 0.11428571 0.12857143 0.14285714 0.15714286 0.17142857 0.18571429 0.2 0.21428571 0.22857143 0.24285714 0.25714286 0.27142857 0.28571429 0.3 0.31428571 0.32857143 0.34285714 0.35714286 0.37142857 0.38571429 0.4 0.41428571 0.42857143 0.44285714 0.45714286 0.47142857 0.48571429 0.5 0.51428571 0.52857143 0.54285714 0.55714286 0.57142857 0.58571429 0.6 0.61428571 0.62857143 0.64285714 0.65714286 0.67142857 0.68571429 0.7 0.71428571 0.72857143 0.74285714 0.75714286 0.77142857 0.78571429 0.8 0.81428571 0.82857143 0.84285714 0.85714286 0.87142857 0.88571429 0.9 0.91428571 0.92857143 0.94285714 0.95714286 0.97142857 0.98571429 1 1 1 1 1 1
  arc A45 (306.7756, -482.5035) -> (308.1344, -472.8354) centre (11.949, -436.1388) ccw
  spline S90 degree 5 poles (308.1344, -472.8354) (308.0565, -472.7849) (307.9007, -472.6841) (307.6668, -472.5335) (307.3547, -472.3335) (306.9638, -472.0852) (306.5724, -471.8385) (306.1803, -471.5934) (305.7877, -471.35) (305.3944, -471.1082) (305.0005, -470.868) (304.6061, -470.6295) (304.211, -470.3927) (303.8153, -470.1576) (303.419, -469.9241) (303.0222, -469.6924) (302.6247, -469.4624) (302.2266, -469.2342) (301.8279, -469.0078) (301.4286, -468.7831) (301.0288, -468.5602) (300.6283, -468.3391) (300.2272, -468.1198) (299.8255, -467.9024) (299.4232, -467.6868) (299.0204, -467.4731) (298.6169, -467.2613) (298.2128, -467.0515) (297.8082, -466.8435) (297.4029, -466.6375) (296.997, -466.4335) (296.5906, -466.2315) (296.1835, -466.0315) (295.7758, -465.8336) (295.3676, -465.6377) (294.9587, -465.4439) (294.5493, -465.2522) (294.1392, -465.0627) (293.7286, -464.8754) (293.3173, -464.6903) (292.9054, -464.5074) (292.493, -464.3268) (292.0799, -464.1484) (291.6662, -463.9724) (291.252, -463.7988) (290.8371, -463.6276) (290.4216, -463.4589) (290.0054, -463.2927) (289.5887, -463.1291) (289.1713, -462.9681) (288.7534, -462.8097) (288.3348, -462.654) (287.9155, -462.5011) (287.4957, -462.3509) (287.0752, -462.2036) (286.6541, -462.0593) (286.2323, -461.9182) (285.8098, -461.7805) (285.3867, -461.646) (284.9629, -461.515) (284.5385, -461.3874) (284.1133, -461.2631) (283.6875, -461.1424) (283.3033, -461.0369) (283.0039, -460.9574) (282.7897, -460.902) (282.6609, -460.8692) (282.6177, -460.8583) knots -1 -1 -1 -1 -1 -1 -0.98571429 -0.97142857 -0.95714286 -0.94285714 -0.92857143 -0.91428571 -0.9 -0.88571429 -0.87142857 -0.85714286 -0.84285714 -0.82857143 -0.81428571 -0.8 -0.78571429 -0.77142857 -0.75714286 -0.74285714 -0.72857143 -0.71428571 -0.7 -0.68571429 -0.67142857 -0.65714286 -0.64285714 -0.62857143 -0.61428571 -0.6 -0.58571429 -0.57142857 -0.55714286 -0.54285714 -0.52857143 -0.51428571 -0.5 -0.48571429 -0.47142857 -0.45714286 -0.44285714 -0.42857143 -0.41428571 -0.4 -0.38571429 -0.37142857 -0.35714286 -0.34285714 -0.32857143 -0.31428571 -0.3 -0.28571429 -0.27142857 -0.25714286 -0.24285714 -0.22857143 -0.21428571 -0.2 -0.18571429 -0.17142857 -0.15714286 -0.14285714 -0.12857143 -0.11428571 -0.10707295 -0.10707295 -0.10707295 -0.10707295 -0.10707295 -0.10707295
  spline S91 degree 3 poles (281.4246, -459.1839) (281.407, -459.3898) (281.4298, -459.5973) (281.5536, -459.9917) (281.6534, -460.175) (281.8923, -460.4624) (282.0187, -460.5732) (282.3013, -460.7513) (282.4557, -460.8174) (282.6177, -460.8583) knots 0 0 0 0 0.062015 0.062015 0.12403 0.12403 0.174133 0.174133 0.224236 0.224236 0.224236 0.224236
  arc A46 (281.4246, -459.1839) -> (282.0094, -450.8217) centre (11.949, -436.1388) ccw
  spline S92 degree 3 poles (283.4238, -449.3296) (283.2183, -449.3518) (283.0191, -449.4139) (282.6557, -449.6111) (282.495, -449.7442) (282.2588, -450.0338) (282.1743, -450.1791) (282.0537, -450.4906) (282.0184, -450.6549) (282.0094, -450.8217) knots 0 0 0 0 0.062015 0.062015 0.12403 0.12403 0.174133 0.174133 0.224236 0.224236 0.224236 0.224236
  spline S93 degree 5 poles (283.4238, -449.3296) (283.4682, -449.3248) (283.6002, -449.3103) (283.8201, -449.2852) (284.1276, -449.2482) (284.5228, -449.1972) (284.9613, -449.1369) (285.3996, -449.073) (285.8377, -449.0057) (286.2756, -448.9349) (286.7133, -448.8607) (287.1508, -448.783) (287.5881, -448.702) (288.0252, -448.6178) (288.4621, -448.5304) (288.8988, -448.4401) (289.3352, -448.347) (289.7714, -448.2511) (290.2074, -448.1524) (290.6431, -448.0511) (291.0785, -447.947) (291.5137, -447.8404) (291.9487, -447.7311) (292.3833, -447.6193) (292.8177, -447.5051) (293.2519, -447.3884) (293.6858, -447.2693) (294.1193, -447.1478) (294.5527, -447.024) (294.9857, -446.8979) (295.4184, -446.7696) (295.8508, -446.639) (296.283, -446.5062) (296.7148, -446.3712) (297.1464, -446.234) (297.5776, -446.0947) (298.0086, -445.9533) (298.4392, -445.8098) (298.8695, -445.6643) (299.2995, -445.5167) (299.7291, -445.3671) (300.1585, -445.2155) (300.5875, -445.0619) (301.0162, -444.9064) (301.4446, -444.7489) (301.8726, -444.5895) (302.3003, -444.4282) (302.7276, -444.265) (303.1546, -444.0999) (303.5813, -443.933) (304.0076, -443.7642) (304.4336, -443.5936) (304.8592, -443.4212) (305.2845, -443.247) (305.7094, -443.071) (306.1339, -442.8932) (306.5581, -442.7137) (306.982, -442.5324) (307.4054, -442.3494) (307.8285, -442.1646) (308.2512, -441.9782) (308.6736, -441.7901) (309.0955, -441.6003) (309.5171, -441.4088) (309.8541, -441.2542) (310.1067, -441.1376) (310.275, -441.0595) (310.3591, -441.0203) knots 0.10707295 0.10707295 0.10707295 0.10707295 0.10707295 0.10707295 0.11428571 0.12857143 0.14285714 0.15714286 0.17142857 0.18571429 0.2 0.21428571 0.22857143 0.24285714 0.25714286 0.27142857 0.28571429 0.3 0.31428571 0.32857143 0.34285714 0.35714286 0.37142857 0.38571429 0.4 0.41428571 0.42857143 0.44285714 0.45714286 0.47142857 0.48571429 0.5 0.51428571 0.52857143 0.54285714 0.55714286 0.57142857 0.58571429 0.6 0.61428571 0.62857143 0.64285714 0.65714286 0.67142857 0.68571429 0.7 0.71428571 0.72857143 0.74285714 0.75714286 0.77142857 0.78571429 0.8 0.81428571 0.82857143 0.84285714 0.85714286 0.87142857 0.88571429 0.9 0.91428571 0.92857143 0.94285714 0.95714286 0.97142857 0.98571429 1 1 1 1 1 1
  arc A47 (310.3591, -441.0203) -> (310.3591, -431.2572) centre (11.949, -436.1388) ccw
  spline S94 degree 5 poles (310.3591, -431.2572) (310.275, -431.2181) (310.1067, -431.14) (309.8541, -431.0233) (309.5171, -430.8688) (309.0955, -430.6773) (308.6736, -430.4875) (308.2512, -430.2993) (307.8285, -430.1129) (307.4054, -429.9282) (306.982, -429.7451) (306.5581, -429.5639) (306.1339, -429.3843) (305.7094, -429.2065) (305.2845, -429.0305) (304.8592, -428.8563) (304.4336, -428.6839) (304.0076, -428.5133) (303.5813, -428.3445) (303.1546, -428.1776) (302.7276, -428.0125) (302.3003, -427.8493) (301.8726, -427.688) (301.4446, -427.5286) (301.0162, -427.3711) (300.5875, -427.2156) (300.1585, -427.062) (299.7291, -426.9104) (299.2995, -426.7608) (298.8695, -426.6132) (298.4392, -426.4677) (298.0086, -426.3242) (297.5776, -426.1828) (297.1464, -426.0435) (296.7148, -425.9064) (296.283, -425.7714) (295.8508, -425.6386) (295.4184, -425.508) (294.9857, -425.3796) (294.5527, -425.2535) (294.1193, -425.1297) (293.6858, -425.0083) (293.2519, -424.8892) (292.8177, -424.7724) (292.3833, -424.6582) (291.9487, -424.5464) (291.5137, -424.4371) (291.0785, -424.3305) (290.6431, -424.2265) (290.2074, -424.1251) (289.7714, -424.0265) (289.3352, -423.9305) (288.8988, -423.8374) (288.4621, -423.7471) (288.0252, -423.6598) (287.5881, -423.5755) (287.1508, -423.4945) (286.7133, -423.4169) (286.2756, -423.3426) (285.8377, -423.2719) (285.3996, -423.2045) (284.9613, -423.1407) (284.5228, -423.0803) (284.1276, -423.0294) (283.8201, -422.9923) (283.6002, -422.9672) (283.4682, -422.9528) (283.4238, -422.948) knots -1 -1 -1 -1 -1 -1 -0.98571429 -0.97142857 -0.95714286 -0.94285714 -0.92857143 -0.91428571 -0.9 -0.88571429 -0.87142857 -0.85714286 -0.84285714 -0.82857143 -0.81428571 -0.8 -0.78571429 -0.77142857 -0.75714286 -0.74285714 -0.72857143 -0.71428571 -0.7 -0.68571429 -0.67142857 -0.65714286 -0.64285714 -0.62857143 -0.61428571 -0.6 -0.58571429 -0.57142857 -0.55714286 -0.54285714 -0.52857143 -0.51428571 -0.5 -0.48571429 -0.47142857 -0.45714286 -0.44285714 -0.42857143 -0.41428571 -0.4 -0.38571429 -0.37142857 -0.35714286 -0.34285714 -0.32857143 -0.31428571 -0.3 -0.28571429 -0.27142857 -0.25714286 -0.24285714 -0.22857143 -0.21428571 -0.2 -0.18571429 -0.17142857 -0.15714286 -0.14285714 -0.12857143 -0.11428571 -0.10707295 -0.10707295 -0.10707295 -0.10707295 -0.10707295 -0.10707295
  spline S95 degree 3 poles (282.0094, -421.4559) (282.0206, -421.6623) (282.072, -421.8645) (282.2495, -422.2379) (282.3739, -422.4055) (282.6504, -422.6568) (282.791, -422.7489) (283.0956, -422.886) (283.2578, -422.93) (283.4238, -422.948) knots 0 0 0 0 0.062015 0.062015 0.12403 0.12403 0.174133 0.174133 0.224236 0.224236 0.224236 0.224236
  arc A48 (282.0094, -421.4559) -> (281.4246, -413.0936) centre (11.949, -436.1388) ccw
  spline S96 degree 3 poles (282.6177, -411.4192) (282.4172, -411.4698) (282.2286, -411.5591) (281.8962, -411.8049) (281.7556, -411.9591) (281.562, -412.2788) (281.4985, -412.4344) (281.4225, -412.7596) (281.4104, -412.9272) (281.4246, -413.0936) knots 0 0 0 0 0.062015 0.062015 0.12403 0.12403 0.174133 0.174133 0.224236 0.224236 0.224236 0.224236
  spline S97 degree 5 poles (282.6177, -411.4192) (282.6609, -411.4083) (282.7897, -411.3756) (283.0039, -411.3202) (283.3033, -411.2406) (283.6875, -411.1352) (284.1133, -411.0144) (284.5385, -410.8901) (284.9629, -410.7625) (285.3867, -410.6315) (285.8098, -410.4971) (286.2323, -410.3593) (286.6541, -410.2182) (287.0752, -410.0739) (287.4957, -409.9267) (287.9155, -409.7765) (288.3348, -409.6235) (288.7534, -409.4678) (289.1713, -409.3094) (289.5887, -409.1484) (290.0054, -408.9848) (290.4216, -408.8186) (290.8371, -408.6499) (291.252, -408.4787) (291.6662, -408.3051) (292.0799, -408.1291) (292.493, -407.9508) (292.9054, -407.7701) (293.3173, -407.5872) (293.7286, -407.4021) (294.1392, -407.2148) (294.5493, -407.0253) (294.9587, -406.8336) (295.3676, -406.6398) (295.7758, -406.4439) (296.1835, -406.246) (296.5906, -406.046) (296.997, -405.844) (297.4029, -405.64) (297.8082, -405.434) (298.2128, -405.2261) (298.6169, -405.0162) (299.0204, -404.8044) (299.4232, -404.5907) (299.8255, -404.3751) (300.2272, -404.1577) (300.6283, -403.9384) (301.0288, -403.7174) (301.4286, -403.4945) (301.8279, -403.2698) (302.2266, -403.0433) (302.6247, -402.8151) (303.0222, -402.5851) (303.419, -402.3534) (303.8153, -402.12) (304.211, -401.8848) (304.6061, -401.648) (305.0005, -401.4095) (305.3944, -401.1693) (305.7877, -400.9275) (306.1803, -400.6841) (306.5724, -400.439) (306.9638, -400.1923) (307.3547, -399.944) (307.6668, -399.7441) (307.9007, -399.5934) (308.0565, -399.4926) (308.1344, -399.4422) knots 0.10707295 0.10707295 0.10707295 0.10707295 0.10707295 0.10707295 0.11428571 0.12857143 0.14285714 0.15714286 0.17142857 0.18571429 0.2 0.21428571 0.22857143 0.24285714 0.25714286 0.27142857 0.28571429 0.3 0.31428571 0.32857143 0.34285714 0.35714286 0.37142857 0.38571429 0.4 0.41428571 0.42857143 0.44285714 0.45714286 0.47142857 0.48571429 0.5 0.51428571 0.52857143 0.54285714 0.55714286 0.57142857 0.58571429 0.6 0.61428571 0.62857143 0.64285714 0.65714286 0.67142857 0.68571429 0.7 0.71428571 0.72857143 0.74285714 0.75714286 0.77142857 0.78571429 0.8 0.81428571 0.82857143 0.84285714 0.85714286 0.87142857 0.88571429 0.9 0.91428571 0.92857143 0.94285714 0.95714286 0.97142857 0.98571429 1 1 1 1 1 1
  arc A49 (308.1344, -399.4422) -> (306.7756, -389.774) centre (11.949, -436.1388) ccw